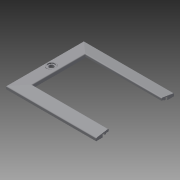
# Autodesk Inventor part: Part1
Saved by Autodesk Inventor 2014 (Build 180170000, 170)
## iProperties
Created: 2017-06-13
Part Number: Part1
Material: Generic
Document SubType Name: Modeling
Designer: resaj
Density: 1 g/cm^3
Appearance: Default
Author: resaj
Autodesk Inventor part; units mm, degrees
sketch "Sketch1" plane through (0, 0, 0) normal (0, 1, 0) x (-1, 0, 0)
  line L0 (0, 34.5) -> (99.3, 34.5)
  line L1 (99.3, 34.5) -> (99.3, 0)
  line L2 (99.3, 0) -> (117.5, 0)
  line L3 (117.5, 0) -> (117.5, 50.75)
  line L4 (117.5, 50.75) -> (0, 50.75)
  line L5 (0, 50.75) -> (0, 34.5)
  line L6 (0, 34.5) -> (0, 0) construction
  line L7 (0, 0) -> (99.3, 0) construction
  dimension "d0" = 117.5
  dimension "d1" = 50.75
  dimension "d3" = 18.2
  dimension "d52" = 34.5
  constraints: 16 end point, 4 parallel, 2 perpendicular, 1 collinear, 1 horizontal
  measures "d0" distance of L3.end L4.end
  measures "d1" distance of L2.end L3.end
  measures "d3" distance of L1.end L2.end
  measures "d52" distance of L0.end L1.end
extrude "Extrusion1" add sketch "Sketch1" along normal blind 6.3
sketch "Sketch2" plane through (0, 0, 50.75) normal (1, 0, 0) x (0, 0, -1)
  line L0 (0, 6.3) -> (16.25, 6.3) projected
  line L1 (0, 0) -> (0, 6.3) projected
  line L2 (0, 3.6) -> (16.25, 6.3)
  point P0 (50.75, 0)
  dimension "d6" = 3.6
  constraints: 2 end point, 1 point on line
  measures "d6" distance of L1.start L2.start
extrude "Extrusion2" cut sketch "Sketch2" against normal through all
sketch "Sketch3" plane through (-99.3, 0, 0) normal (0, 0, -1) x (-1, 0, 0)
  line L0 (18.2, 0) -> (18.2, 6.3) projected
  line L1 (0, 6.3) -> (18.2, 6.3) projected
  line L2 (0, 6.3) -> (18.2, 3.6)
  point P0 (-99.3, 0)
  dimension "d9" = 3.6
  constraints: 2 end point, 1 point on line
  measures "d9" distance of L0.start L2.end
extrude "Extrusion3" cut sketch "Sketch3" against normal through all
sketch "Sketch4" plane through (0, 0, 50.75) normal (1, 0, 0) x (0, 0, -1)
  line L0 (16.25, 6.3) -> (0, 3.6) projected
  line L1 (0, 0) -> (0, 3.6) projected
  line L2 (0, 0) -> (16.25, 0) projected
  line L3 (16.25, 0) -> (16.25, 6.3) projected
  line L4 (16.25, 2.75) -> (12.75, 2.75) construction
  line L5 (12.75, 2.75) -> (12.75, 1.1) construction
  line L6 (10.85, 1.1) -> (10.85, 4.4) construction
  line L7 (10.85, 4.4) -> (1.5, 2.8465)
  line L8 (1.5, 2.8465) -> (1.5, 0)
  line L9 (10.85, 1.1) -> (12.75, 1.1) construction
  line L10 (10.85, 1.1) -> (10.85, 0) construction
  line L11 (10.85, 4.4) -> (16.25, 5.2972)
  point P0 (50.75, 0)
  dimension "d12" = 1.5
  dimension "d14" = 3.5
  dimension "d15" = 3.55
  dimension "d17" = 1.9
  dimension "d18" = 3.3
  dimension "d19" = 1.65
  constraints: 16 end point, 5 perpendicular, 4 point on line, 2 parallel, 1 collinear
  measures "d12" distance between parallel lines of L1 L8
  measures "d14" distance of L4.start L4.end
  measures "d15" distance from line of L4 L0.start
  measures "d17" distance between parallel lines of L5 L6
  measures "d18" distance of L6.start L6.end
  measures "d19" distance of L4.end L5.end
ref_plane "Work Plane1" through (-99.3, 6.3, 34.5) normal (0.6660158, 0, 0.7459377) x (-0.7414119, -0.1099897, 0.6619749)
extrude "Extrusion4" cut sketch "Sketch4" against normal up to surface contours L3 L2 L8 L7 L11 surface through (-99.3, 6.3, 34.5) normal (0.6660158, 0, 0.7459377)
sketch "Sketch5" plane through (-99.3, 0, 0) normal (0, 0, -1) x (-1, 0, 0)
  line L0 (16.52, 2.8465) -> (0, 5.2972) projected
  line L1 (16.52, 0) -> (16.52, 2.8465) projected
  line L2 (0, 0) -> (16.52, 0) projected
  line L3 (0, 0) -> (0, 5.2972) projected
  point P0 (-99.3, 0)
extrude "Extrusion5" cut sketch "Sketch5" against normal up to surface surface through (-99.3, 6.3, 34.5) normal (0.6660158, 0, 0.7459377)
sketch "Sketch6" plane through (0, 0, 0) normal (0, -1, 0) x (1, 0, 0)
  line L0 (-115.82, 49.25) -> (0, 49.25) projected
  line L1 (-115.82, 0) -> (-117.5, 0) projected
  line L2 (-71.975, 49.25) -> (-71.975, 42.45)
  line L3 (-71.975, 42.45) -> (-69.325, 42.45)
  line L4 (-69.325, 42.45) -> (-69.325, 49.25)
  line L5 (-1.325, 49.25) -> (-1.325, 42.45)
  line L6 (-1.325, 42.45) -> (0, 42.45)
  line L7 (0, 42.45) -> (0, 49.25)
  point P0 (0, 0)
  dimension "d27" = 2.65
  dimension "d28" = 1.325
  dimension "d29" = 6.8
  dimension "d30" = 68
  constraints: 12 end point, 4 perpendicular, 3 parallel, 3 point on line
  measures "d27" distance of L2.end L3.end
  measures "d28" distance of L5.end L6.end
  measures "d29" distance of L5.start L5.end
  measures "d30" distance between parallel lines of L5 L4
extrude "Extrusion6" add sketch "Sketch6" against normal up to surface surface through (0, 2.8465, 49.25) normal (0, 0.9864758, 0.1639068)
fillet "Fillet1" radius 1 3 edges at (-1.325, 1.9882, 42.45) (-69.325, 1.9882, 42.45) (-71.975, 1.9882, 42.45)
ref_plane "Work Plane2" through (0, 1.6, 0) normal (0, -1, 0) x (1, 0, 0)
sketch "Sketch7" plane through (0, 1.6, 0) normal (0, -1, 0) x (1, 0, 0)
  arc A0 (-1.325, 43.45) -> (-0.325, 42.45) centre (-0.325, 43.45) ccw projected
  line L0 (-1.325, 43.45) -> (-1.325, 49.25) projected
  line L1 (-1.325, 49.25) -> (-69.325, 49.25) projected
  line L2 (-69.325, 49.25) -> (-69.325, 43.45) projected
  arc A1 (-70.325, 42.45) -> (-69.325, 43.45) centre (-70.325, 43.45) ccw projected
  line L3 (-70.325, 42.45) -> (-70.975, 42.45) projected
  arc A2 (-71.975, 43.45) -> (-70.975, 42.45) centre (-70.975, 43.45) ccw projected
  line L4 (-71.975, 43.45) -> (-71.975, 49.25) projected
  line L5 (-71.975, 49.25) -> (-115.82, 49.25) projected
  line L6 (-115.82, 49.25) -> (-115.82, 0) projected
  line L7 (-115.82, 0) -> (-117.5, 0) projected
  line L8 (-117.5, 0) -> (-117.5, 50.75) projected
  line L9 (-117.5, 50.75) -> (0, 50.75) projected
  line L10 (0, 50.75) -> (0, 42.45) projected
  line L11 (0, 42.45) -> (-0.325, 42.45) projected
  line L12 (-115.82, 49.25) -> (-99.3, 34.5) projected
  line L13 (-115.82, 0) -> (-115.82, 49.25) projected
  line L14 (-99.3, 0) -> (-115.82, 0) projected
  line L15 (-99.3, 34.5) -> (-99.3, 0) projected
  line L16 (-115.82, 7) -> (-99.3, 7)
  point P0 (0, 0)
  dimension "d35" = 7
  constraints: 2 end point, 2 point on line, 1 perpendicular
  measures "d35" distance between parallel lines of L16 L14
extrude "Extrusion7" add sketch "Sketch7" against normal up to surface contours L6 L16 L15 L14 surface through (-99.3, 5.2972, 0) normal (-0.1467456, 0.9891743, 0)
sketch "Sketch8" plane through (0, 1.6, 0) normal (0, -1, 0) x (1, 0, 0)
  line L0 (-115.82, 0) -> (-99.3, 0) projected
  circle A0 centre (-109, 0) radius 3
  arc A1 (-71.975, 43.45) -> (-70.975, 42.45) centre (-70.975, 43.45) ccw projected
  line L1 (-70.975, 42.45) -> (-70.325, 42.45) projected
  arc A2 (-70.325, 42.45) -> (-69.325, 43.45) centre (-70.325, 43.45) ccw projected
  line L2 (-69.325, 43.45) -> (-69.325, 49.25) projected
  line L3 (-69.325, 49.25) -> (-1.325, 49.25) projected
  line L4 (-1.325, 49.25) -> (-1.325, 43.45) projected
  arc A3 (-1.325, 43.45) -> (-0.325, 42.45) centre (-0.325, 43.45) ccw projected
  line L5 (-0.325, 42.45) -> (0, 42.45) projected
  line L6 (0, 50.75) -> (0, 42.45) projected
  line L7 (-117.5, 50.75) -> (0, 50.75) projected
  line L8 (-117.5, 0) -> (-117.5, 50.75) projected
  line L9 (-115.82, 0) -> (-117.5, 0) projected
  line L10 (-115.82, 0) -> (-115.82, 49.25) projected
  line L11 (-115.82, 49.25) -> (-71.975, 49.25) projected
  line L12 (-71.975, 49.25) -> (-71.975, 43.45) projected
  point P0 (-100.7, 0)
  point P1 (0, 0)
  dimension "d39" = 6
  dimension "d40" = 8.5
  constraints: 1 centre point, 1 point on line
  measures "d39" diameter of A0
  measures "d40" distance from line of A0.centre L8
extrude "Extrusion8" cut sketch "Sketch8" against normal through all contours A0 L0 | L0 A0
sketch "Sketch9" plane through (0, 1.6, 0) normal (0, -1, 0) x (1, 0, 0)
  line L0 (-99.3, 7) -> (-115.82, 7) projected
  line L1 (-115.82, 0) -> (-115.82, 7) projected
  line L2 (-115.82, 0) -> (-112, 0) projected
  line L3 (-115.82, 5.3) -> (-109.32, 5.3)
  line L4 (-109.32, 5.3) -> (-109.32, 7)
  point P0 (0, 0)
  dimension "d44" = 6.5
  dimension "d45" = 1.7
  constraints: 4 end point, 2 point on line, 1 parallel, 1 perpendicular
  measures "d44" distance of L3.start L3.end
  measures "d45" distance of L3.end L4.end
extrude "Extrusion9" add sketch "Sketch9" along normal blind 0.8
ref_plane "Work Plane3" through (0, 1.7, 0) normal (0, -1, 0) x (1, 0, 0)
sketch "Sketch10" plane through (0, 1.7, 0) normal (0, -1, 0) x (1, 0, 0)
  line L0 (-99.3, 34.5) -> (-99.3, 7) projected
  line L1 (0, 34.5) -> (-99.3, 34.5) projected
  line L2 (0, 42.45) -> (0, 34.5) projected
  line L3 (-99.3, 7) -> (-109.32, 7) projected
  line L4 (-101.3, 39.7) -> (-101.3, 7)
  line L5 (-101.3, 39.7) -> (0, 39.7)
  line L6 (0, 37.7) -> (-99.3, 37.7)
  line L7 (-106, 0) -> (-99.3, 0) projected
  line L8 (-99.3, 34.5) -> (-99.3, 37.7)
  point P0 (0, 0)
  dimension "d49" = 2
  dimension "d53" = 39.7
  dimension "d54" = 2
  constraints: 8 end point, 3 parallel, 3 point on line, 2 perpendicular, 1 collinear
  measures "d49" distance between parallel lines of L5 L6
  measures "d53" distance between parallel lines of L5 L7
  measures "d54" distance between parallel lines of L0 L4
extrude "Extrusion10" add sketch "Sketch10" against normal blind 3.7 contours L0 L3 L4 L5 L2 L6 L8
ref_plane "Work Plane4" through (0, 2.95, 0) normal (0, -1, 0) x (1, 0, 0)
sketch "Sketch11" plane through (0, 2.95, 0) normal (0, -1, 0) x (1, 0, 0)
  line L0 (0, 37.7) -> (-99.3, 37.7) projected
  line L1 (-99.3, 37.7) -> (-99.3, 34.5) projected
  line L2 (0, 34.5) -> (-99.3, 34.5) projected
  line L3 (0, 37.7) -> (0, 34.5) projected
  point P0 (0, 0)
extrude "Extrusion11" add sketch "Sketch11" against normal up to surface surface through (0, 2.8465, 49.25) normal (0, 0.9864758, 0.1639068)
ref_plane "Work Plane5" through (0, 5.8, 0) normal (0, -1, 0) x (1, 0, 0)
sketch "Sketch12" plane through (0, 5.8, 0) normal (0, -1, 0) x (1, 0, 0)
  arc A0 (-106, 0) -> (-112, 0) centre (-109, 0) ccw projected
  line L0 (-117.5, 0) -> (-112, 0) projected
  line L1 (-117.5, 50.75) -> (-117.5, 0) projected
  line L2 (-99.3, 34.5) -> (-117.5, 50.75) projected
  line L3 (-99.3, 34.5) -> (-99.3, 0) projected
  line L4 (-106, 0) -> (-99.3, 0) projected
  arc A1 (-104.5, 0) -> (-113.5, 0) centre (-109, 0) ccw
  arc A2 (-102.9, 0) -> (-115.1, 0) centre (-109, 0) ccw
  point P0 (0, 0)
  dimension "d61" = 4.5
  dimension "d62" = 6.1
  constraints: 4 point on circle, 4 point on line, 2 centre point, 2 coincident
  measures "d61" radius of A1
  measures "d62" radius of A2
extrude "Extrusion12" add sketch "Sketch12" against normal up to surface contours A1 L0 A2 L4 surface through (-117.5, 3.6, 0) normal (0.1467456, -0.9891743, 0)
sketch "Sketch13" plane through (0, 5.8, 0) normal (0, 1, 0) x (1, 0, 0)
  arc A0 (-113.5, 0) -> (-104.5, 0) centre (-109, 0) ccw projected
  line L0 (-115.1, 0) -> (-113.5, 0) projected
  line L1 (-113.5, 0) -> (-104.5, 0)
  point P0 (0, 0)
  constraints: 2 end point, 1 collinear
extrude "Extrusion13" cut sketch "Sketch13" against normal blind 1.35
mirror "Mirror1" about plane through (-99.3, 0, 0) normal (0, 0, -1)
fillet "Fillet2" radius 1 7 edges at (-49.65, 6.3, -34.5) (-99.3, 6.3, 0) (-49.65, 6.3, 34.5) (-58.75, 3.6, 50.75) (-58.75, 3.6, -50.75) (-117.5, 3.6, 25.375) (-117.5, 3.6, -25.375)
fillet "Fillet3" radius 1 2 edges at (-109, 5.8, 6.1) (-109, 5.8, -6.1)
body "Solid1"
